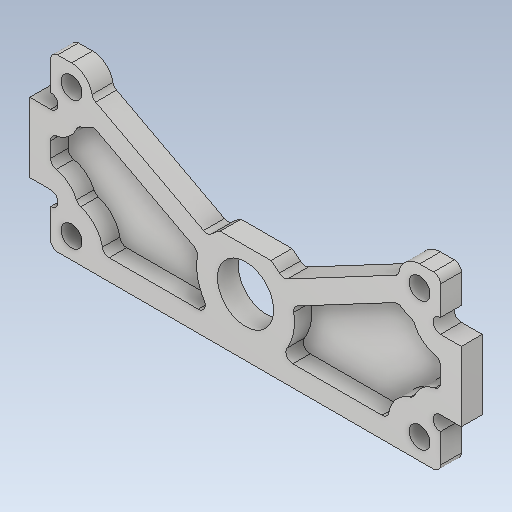
# Autodesk Inventor part: 横回転フレーム２
Saved by Autodesk Inventor 2020 (Build 240168000, 168)
## iProperties
Created: 2019-09-04
Part Number: 横回転フレーム２
Material: アルミニウム 2014-T4
Document SubType Name: Modeling
Designer: tanjihayato
Density: 2.8 g/cm^3
Appearance: サテン
Mass: 5.33751 g
Surface Area: 30.1878 cm^2
Volume: 1.90625 cm^3
Author: tanjihayato
Autodesk Inventor part; units mm, degrees
ref_plane "YZ Plane" through (0, 0, 0) normal (1, 0, 0) x (0, 1, 0)
ref_plane "XZ Plane" through (0, 0, 0) normal (0, 1, 0) x (-1, 0, 0)
ref_plane "XY Plane" through (0, 0, 0) normal (0, 0, 1) x (1, 0, 0)
sketch "スケッチ1" plane through (0, 0, 0) normal (0, 0, 1) x (1, 0, 0)
  line L0 (0, 0) -> (0, 4) construction
  line L1 (0, 0) -> (-5.3121, 14.0279)
  line L2 (-5.3121, 14.0279) -> (3.582, -2.7619)
  circle A0 centre (0.3052, 3.4238) radius 4
  line L3 (-57.3278, -140) -> (69.8706, -140)
  line L4 (0.3052, 3.4238) -> (-114.5721, -57.4302)
  circle A1 centre (0, 0) radius 23.1
  circle A2 centre (0, -29.1039) radius 6.0039
  line L5 (0, 0) -> (0, -29.1039) construction
  circle A3 centre (0, -29.1039) radius 20.05
  circle A4 centre (0, -4.0039) radius 5.05
  circle A5 centre (0, 4) radius 3
  circle A6 centre (0, -4.0039) radius 20.05
  circle A7 centre (-14, 13.4079) radius 2.2921
  circle A8 centre (14, 13.4079) radius 2.2921
  circle A9 centre (14, -21.4157) radius 2.2921
  circle A10 centre (-14, -21.4157) radius 2.2921
  circle A11 centre (-14, 13.4079) radius 14
  circle A12 centre (14, 13.4079) radius 14
  circle A13 centre (14, -21.4157) radius 14
  circle A14 centre (-14, -21.4157) radius 14
  line L6 (-14, 13.4079) -> (-14, -21.4157) construction
  line L7 (-14, -21.4157) -> (14, -21.4157) construction
  circle A15 centre (0, 0) radius 9
  line L8 (3.582, -2.7619) -> (-0.1629, 4.3075) construction
  line L9 (6.2551, -1.3458) -> (2.5102, 5.7235)
  line L10 (-2.836, 2.8915) -> (0.9089, -4.1779)
  arc A16 (0.9089, -4.1779) -> (6.2551, -1.3458) centre (3.582, -2.7619) ccw
  arc A17 (2.5102, 5.7235) -> (-2.836, 2.8915) centre (-0.1629, 4.3075) ccw
  line L11 (-5, 2.8868) -> (5, 2.8868) construction
  line L12 (5, 2.8868) -> (0, -5.7735) construction
  line L13 (0, -5.7735) -> (-5, 2.8868) construction
  circle A18 centre (-5, 2.8868) radius 1.5
  circle A19 centre (5, 2.8868) radius 1.5
  circle A20 centre (0, -5.7735) radius 1.5
  line L14 (-28, 26.018) -> (-28, -39.908)
  line L15 (28, 26.019) -> (28, -39.909)
  line L16 (-28, 29.3694) -> (28, 29.3694)
  circle A21 centre (0, 0) radius 25.1
  line L17 (-28, -18.848) -> (28, -18.848)
  circle A22 centre (0, -29.1039) radius 8.0039
  circle A23 centre (-25, 26.3694) radius 3
  circle A24 centre (25, 26.3694) radius 3
  circle A25 centre (25, -34.3772) radius 3
  circle A26 centre (-25, -34.3772) radius 3
  circle A27 centre (-25, -15.848) radius 3
  circle A28 centre (25, -15.848) radius 3
  circle A29 centre (-25, -15.848) radius 4.5
  circle A30 centre (25, -15.848) radius 4.5
  circle A31 centre (0, -4.0039) radius 4.5
  point P0 (1.7095, 0.7728)
  dimension "d0" = 4
  dimension "d1" = 15
  dimension "d2" = 11.348
  dimension "d3" = 19
  dimension "d4" = 8
  dimension "d5" = 12
  dimension "d6" = 140
  dimension "d7" = 130
  dimension "d8" = 46.2
  dimension "d9" = 29.1039
  dimension "d10" = 40.1
  dimension "d11" = 10.1
  dimension "d12" = 6
  dimension "d13" = 40.1
  dimension "d14" = 22.3421
  dimension "d15" = 22.3421
  dimension "d16" = 22.3421
  dimension "d17" = 22.3421
  dimension "d18" = 28
  dimension "d19" = 28
  dimension "d20" = 28
  dimension "d21" = 28
  dimension "d22" = 18
  dimension "d23" = 8
  dimension "d24" = 6.05
  dimension "d25" = 3
  dimension "d26" = 3
  dimension "d27" = 3
  dimension "d28" = 10
  dimension "d29" = 2
  dimension "d30" = 2
  dimension "d31" = 6
  dimension "d32" = 6
  dimension "d33" = 6
  dimension "d34" = 6
  dimension "d35" = 6
  dimension "d36" = 6
  dimension "d37" = 9
  dimension "d38" = 9
  dimension "d39" = 9
  constraints: 38 end point, 32 centre point, 28 tangent, 16 coincident, 8 point on line, 5 vertical, 4 point on circle, 3 horizontal, 3 perpendicular, 1 midpoint, 1 parallel, 7 other
  measures "d0" distance of L0.start L0.end
  measures "d1" distance of L0.start L1.end
  measures "d2" distance of L0.end L1.end
  measures "d3" distance of L1.end L2.end
  measures "d4" diameter of A0
  measures "d5" distance of L1.end L4.start
  measures "d6" distance from line of L3 L0.start
  measures "d7" distance of L4.start L4.end
  measures "d8" diameter of A1
  measures "d9" distance of L5.end L0.start
  measures "d10" diameter of A3
  measures "d11" diameter of A4
  measures "d12" diameter of A5
  measures "d13" diameter of A6
  measures "d14" distance of A7.centre A6.centre
  measures "d15" distance of A4.centre A8.centre
  measures "d16" distance of A4.centre A9.centre
  measures "d17" distance of A4.centre A10.centre
  measures "d18" diameter of A11
  measures "d19" diameter of A12
  measures "d20" diameter of A13
  measures "d21" diameter of A14
  measures "d22" diameter of A15
  measures "d23" distance of L2.end L8.end
  measures "d24" diameter of A17
  measures "d25" diameter of A18
  measures "d26" diameter of A19
  measures "d27" diameter of A20
  measures "d28" distance of L11.end L12.end
  measures "d29" radial gap between concentric circles of A1 A21
  measures "d30" radial gap between concentric circles of A2 A22
  measures "d31" diameter of A23
  measures "d32" diameter of A24
  measures "d33" diameter of A25
  measures "d34" diameter of A26
  measures "d35" diameter of A27
  measures "d36" diameter of A28
  measures "d37" diameter of A29
  measures "d38" diameter of A30
  measures "d39" diameter of A31
sketch "スケッチ2" plane through (0, 0, 0) normal (0, 0, 1) x (1, 0, 0)
  circle A0 centre (-25, -15.848) radius 3 construction
  circle A1 centre (-25, -34.3772) radius 3 construction
  circle A2 centre (25, -34.3772) radius 3 construction
  circle A3 centre (25, -15.848) radius 3 construction
  circle A4 centre (0, -29.1039) radius 20.05 construction
  circle A5 centre (-25, -15.848) radius 1.5
  circle A6 centre (25, -15.848) radius 1.5
  circle A7 centre (25, -34.3772) radius 1.5
  circle A8 centre (-25, -34.3772) radius 1.5
  circle A9 centre (0, -29.1039) radius 4.025
  line L0 (-28, -37.3772) -> (28, -37.3772)
  line L1 (28, -37.3772) -> (28, -32.2126)
  line L2 (28, -30.1126) -> (31, -30.1126)
  line L3 (31, -30.1126) -> (31, -20.1126)
  line L4 (31, -20.1126) -> (28, -20.1126)
  line L5 (28, -18.0126) -> (28, -12.848)
  line L6 (28, -12.848) -> (-28, -12.848)
  line L7 (-28, -12.848) -> (-28, -18.0126)
  line L8 (-28, -20.1126) -> (-31, -20.1126)
  line L9 (-31, -20.1126) -> (-31, -30.1126)
  line L10 (-31, -30.1126) -> (-28, -30.1126)
  line L11 (-28, -32.2126) -> (-28, -37.3772)
  arc A10 (-28, -32.2126) -> (-28, -30.1126) centre (-28, -31.1626) ccw
  arc A11 (-28, -20.1126) -> (-28, -18.0126) centre (-28, -19.0626) ccw
  arc A12 (28, -18.0126) -> (28, -20.1126) centre (28, -19.0626) ccw
  arc A13 (28, -30.1126) -> (28, -32.2126) centre (28, -31.1626) ccw
  line L12 (28, -23.1126) -> (28, -27.1126)
  arc A14 (28, -27.1126) -> (24.1322, -29.9617) centre (28, -31.1626) ccw
  line L13 (-28, -27.1126) -> (-28, -23.1126)
  arc A15 (-28, -23.1126) -> (-24.1322, -20.2636) centre (-28, -19.0626) ccw
  arc A16 (20.5, -15.848) -> (24.1322, -20.2636) centre (25, -15.848) ccw
  arc A17 (24.1322, -29.9617) -> (20.5, -34.3772) centre (25, -34.3772) ccw
  arc A18 (-20.5, -34.3772) -> (-24.1322, -29.9617) centre (-25, -34.3772) ccw
  arc A19 (-24.1322, -20.2636) -> (-20.5, -15.848) centre (-25, -15.848) ccw
  arc A20 (-24.1322, -29.9617) -> (-28, -27.1126) centre (-28, -31.1626) ccw
  arc A21 (24.1322, -20.2636) -> (28, -23.1126) centre (28, -19.0626) ccw
  arc A22 (4.6415, -34.3772) -> (-4.6415, -34.3772) centre (0, -29.1039) ccw
  line L14 (20.5, -34.3772) -> (4.6415, -34.3772)
  line L15 (-4.6415, -34.3772) -> (-20.5, -34.3772)
  line L16 (-25, -15.848) -> (0, -29.1039) construction
  arc A23 (-24.2973, -14.5228) -> (-25.7027, -17.1733) centre (-25, -15.848) ccw
  arc A24 (-0.7027, -30.4291) -> (0.7027, -27.7787) centre (0, -29.1039) ccw
  line L17 (25, -15.848) -> (0, -29.1039) construction
  arc A25 (25.7027, -17.1733) -> (24.2973, -14.5228) centre (25, -15.848) ccw
  arc A26 (-0.7027, -27.7787) -> (0.7027, -30.4291) centre (0, -29.1039) ccw
  line L18 (0.7027, -30.4291) -> (4.0026, -28.6794)
  line L19 (2.5972, -26.029) -> (-0.7027, -27.7787)
  line L20 (0.7027, -27.7787) -> (-2.5972, -26.029)
  line L21 (-4.0026, -28.6794) -> (-0.7027, -30.4291)
  line L22 (-5.3607, -24.5637) -> (-20.549, -16.5103)
  line L23 (-22.0019, -15.7399) -> (-24.2973, -14.5228)
  line L24 (-25.7027, -17.1733) -> (-23.4073, -18.3903)
  line L25 (-21.9544, -19.1607) -> (-6.766, -27.2141)
  line L26 (6.766, -27.2141) -> (21.9544, -19.1607)
  line L27 (23.4073, -18.3903) -> (25.7027, -17.1733)
  line L28 (24.2973, -14.5228) -> (21.798, -15.848)
  line L29 (20.549, -16.5103) -> (5.3607, -24.5637)
  line L30 (-20.5, -15.848) -> (20.5, -15.848)
  line L31 (21.798, -15.848) -> (22, -15.848)
  point P0 (0, 0)
  point P1 (-12.5, -22.476)
  point P2 (12.5, -22.476)
  dimension "d40" = 3
  dimension "d41" = 3
  dimension "d42" = 3
  dimension "d43" = 3
  dimension "d44" = 8.05
  dimension "d47" = 3
  dimension "d48" = 10
  dimension "d49" = 3
  dimension "d50" = 3
  dimension "d51" = 10
  dimension "d52" = 7.2646
  dimension "d53" = 7.2646
  dimension "d54" = 2.1
  dimension "d55" = 2.1
  dimension "d56" = 2.1
  dimension "d57" = 2.1
  dimension "d59" = 3
  dimension "d60" = 3
  dimension "d61" = 3
  dimension "d62" = 3
  dimension "d64" = 3
  dimension "d66" = 3
  dimension "d67" = 4.05
  dimension "d68" = 4.05
  dimension "d69" = 4.05
  dimension "d70" = 4.05
  dimension "d71" = 3
  dimension "d72" = 3
  dimension "d73" = 3
  dimension "d74" = 3
  dimension "d75" = 3
  constraints: 68 end point, 50 point on circle, 32 tangent, 22 centre point, 18 parallel, 9 point on line, 6 perpendicular, 5 coincident, 2 horizontal, 2 midpoint, 1 concentric, 1 vertical
  measures "d40" diameter of A5
  measures "d41" diameter of A6
  measures "d42" diameter of A7
  measures "d43" diameter of A8
  measures "d44" diameter of A9
  measures "d47" distance of L2.start L2.end
  measures "d48" distance of L2.end L3.end
  measures "d49" distance of L3.end L4.end
  measures "d50" distance of L8.start L8.end
  measures "d51" distance of L8.end L9.end
  measures "d52" distance between parallel lines of L4 L6
  measures "d53" distance between parallel lines of L0 L2
  measures "d54" diameter of A10
  measures "d55" diameter of A11
  measures "d56" diameter of A12
  measures "d57" diameter of A13
  measures "d59" radial gap between concentric circles of A6 A16
  measures "d60" radial gap between concentric circles of A7 A17
  measures "d61" radial gap between concentric circles of A8 A18
  measures "d62" radial gap between concentric circles of A5 A19
  measures "d64" distance between parallel lines of L3 L12
  measures "d66" distance between parallel lines of L9 L13
  measures "d67" radius of A15
  measures "d68" radius of A20
  measures "d69" radius of A14
  measures "d70" radius of A21
  measures "d71" radial gap between concentric circles of A9 A22
  measures "d72" distance between parallel lines of L0 L14
  measures "d73" distance between parallel lines of L0 L15
  measures "d74" diameter of A24
  measures "d75" diameter of A26
extrude "押し出し1" add sketch "スケッチ2" along normal blind 3 contours L11 A10 L10 L9 L8 A11 L7 L6 L5 A12 L4 L3 L2 A13 L1 L0 | L26 A22 L29 A16 | A22 L25 A19 L22
fillet "フィレット1" radius 1 22 edges at (-28, -23.1126, 1.5) (-28, -27.1126, 1.5) (-24.1322, -29.9617, 1.5) (-20.5, -34.3772, 1.5) (-4.6415, -34.3772, 1.5) (-6.766, -27.2141, 1.5) (-21.9544, -19.1607, 1.5) (-24.1322, -20.2636, 1.5) (28, -27.1126, 1.5) (28, -23.1126, 1.5) (24.1322, -20.2636, 1.5) (21.9544, -19.1607, 1.5) (6.766, -27.2141, 1.5) (4.6415, -34.3772, 1.5) (20.5, -34.3772, 1.5) (24.1322, -29.9617, 1.5) (20.5, -15.848, 1.5) (-20.5, -15.848, 1.5) (-20.549, -16.5103, 1.5) (-5.3607, -24.5637, 1.5) (5.3607, -24.5637, 1.5) (20.549, -16.5103, 1.5)
sketch "スケッチ3" plane through (0, 0, 0) normal (0, 0, -1) x (-1, 0, 0)
  line L0 (-17.7774, -15.848) -> (17.7774, -15.848) projected
  arc A0 (18.2458, -17.7315) -> (17.7774, -15.848) centre (17.7774, -16.848) ccw projected
  line L1 (18.2458, -17.7315) -> (6.0345, -24.2064) projected
  arc A1 (4.8724, -24.0433) -> (6.0345, -24.2064) centre (5.566, -23.3229) ccw projected
  arc A2 (4.8724, -24.0433) -> (-4.8724, -24.0433) centre (0, -29.1039) ccw projected
  arc A3 (-6.0345, -24.2064) -> (-4.8724, -24.0433) centre (-5.566, -23.3229) ccw projected
  line L2 (-6.0345, -24.2064) -> (-18.2458, -17.7315) projected
  arc A4 (-17.7774, -15.848) -> (-18.2458, -17.7315) centre (-17.7774, -16.848) ccw projected
  line L3 (28, -24.0126) -> (28, -26.2126) projected
  arc A5 (27.198, -27.1928) -> (28, -26.2126) centre (27, -26.2126) ccw projected
  arc A6 (27.198, -27.1928) -> (24.2958, -29.5251) centre (28, -31.1626) ccw projected
  arc A7 (23.6755, -30.0765) -> (24.2958, -29.5251) centre (23.3812, -29.1208) ccw projected
  arc A8 (23.6755, -30.0765) -> (20.575, -33.559) centre (25, -34.3772) ccw projected
  arc A9 (19.5917, -34.3772) -> (20.575, -33.559) centre (19.5917, -33.3772) ccw projected
  line L4 (19.5917, -34.3772) -> (6.7926, -34.3772) projected
  arc A10 (5.9462, -32.8447) -> (6.7926, -34.3772) centre (6.7926, -33.3772) ccw projected
  arc A11 (5.9462, -32.8447) -> (6.9228, -27.9103) centre (0, -29.1039) ccw projected
  arc A12 (7.4399, -26.8568) -> (6.9228, -27.9103) centre (7.9083, -27.7403) ccw projected
  line L5 (7.4399, -26.8568) -> (21.3745, -19.4682) projected
  arc A13 (22.417, -19.5329) -> (21.3745, -19.4682) centre (21.843, -20.3517) ccw projected
  arc A14 (22.417, -19.5329) -> (23.6755, -20.1487) centre (25, -15.848) ccw projected
  arc A15 (24.2958, -20.7001) -> (23.6755, -20.1487) centre (23.3812, -21.1044) ccw projected
  arc A16 (24.2958, -20.7001) -> (27.198, -23.0324) centre (28, -19.0626) ccw projected
  arc A17 (28, -24.0126) -> (27.198, -23.0324) centre (27, -24.0126) ccw projected
  line L6 (-28, -26.2126) -> (-28, -24.0126) projected
  arc A18 (-27.198, -23.0324) -> (-28, -24.0126) centre (-27, -24.0126) ccw projected
  arc A19 (-27.198, -23.0324) -> (-24.2958, -20.7001) centre (-28, -19.0626) ccw projected
  arc A20 (-23.6755, -20.1487) -> (-24.2958, -20.7001) centre (-23.3812, -21.1044) ccw projected
  arc A21 (-23.6755, -20.1487) -> (-22.417, -19.5329) centre (-25, -15.848) ccw projected
  arc A22 (-21.3745, -19.4682) -> (-22.417, -19.5329) centre (-21.843, -20.3517) ccw projected
  line L7 (-21.3745, -19.4682) -> (-7.4399, -26.8568) projected
  arc A23 (-6.9228, -27.9103) -> (-7.4399, -26.8568) centre (-7.9083, -27.7403) ccw projected
  arc A24 (-6.9228, -27.9103) -> (-5.9462, -32.8447) centre (0, -29.1039) ccw projected
  arc A25 (-6.7926, -34.3772) -> (-5.9462, -32.8447) centre (-6.7926, -33.3772) ccw projected
  line L8 (-6.7926, -34.3772) -> (-19.5917, -34.3772) projected
  arc A26 (-20.575, -33.559) -> (-19.5917, -34.3772) centre (-19.5917, -33.3772) ccw projected
  arc A27 (-20.575, -33.559) -> (-23.6755, -30.0765) centre (-25, -34.3772) ccw projected
  arc A28 (-24.2958, -29.5251) -> (-23.6755, -30.0765) centre (-23.3812, -29.1208) ccw projected
  arc A29 (-24.2958, -29.5251) -> (-27.198, -27.1928) centre (-28, -31.1626) ccw projected
  arc A30 (-28, -26.2126) -> (-27.198, -27.1928) centre (-27, -26.2126) ccw projected
  circle A31 centre (0, -29.1039) radius 4.025 projected
  line L9 (-28, -37.3772) -> (28, -37.3772) projected
  line L10 (28, -37.3772) -> (28, -32.2126) projected
  arc A32 (28, -30.1126) -> (28, -32.2126) centre (28, -31.1626) ccw projected
  line L11 (28, -30.1126) -> (31, -30.1126) projected
  line L12 (31, -30.1126) -> (31, -20.1126) projected
  line L13 (31, -20.1126) -> (28, -20.1126) projected
  arc A33 (28, -18.0126) -> (28, -20.1126) centre (28, -19.0626) ccw projected
  line L14 (28, -18.0126) -> (28, -12.848) projected
  line L15 (28, -12.848) -> (-28, -12.848) projected
  line L16 (-28, -12.848) -> (-28, -18.0126) projected
  arc A34 (-28, -20.1126) -> (-28, -18.0126) centre (-28, -19.0626) ccw projected
  line L17 (-28, -20.1126) -> (-31, -20.1126) projected
  line L18 (-31, -20.1126) -> (-31, -30.1126) projected
  line L19 (-31, -30.1126) -> (-28, -30.1126) projected
  arc A35 (-28, -32.2126) -> (-28, -30.1126) centre (-28, -31.1626) ccw projected
  line L20 (-28, -32.2126) -> (-28, -37.3772) projected
  circle A36 centre (25, -15.848) radius 1.5 projected
  circle A37 centre (-25, -15.848) radius 1.5 projected
  circle A38 centre (-25, -34.3772) radius 1.5 projected
  circle A39 centre (25, -34.3772) radius 1.5 projected
  point P0 (0, 0)
extrude "押し出し2" add sketch "スケッチ3" against normal blind 0.5 contours L0 A0 L1 A1 A2 A3 L2 A4 | L3 A5 A6 A7 A8 A9 L4 A10 A11 A12 L5 A13 A14 A15 A16 A17 | L6 A18 A19 A20 A21 A22 L7 A23 A24 A25 L8 A26 A27 A28 A29 A30
sketch "スケッチ4" plane through (0, 0, 3) normal (0, 0, 1) x (1, 0, 0)
  line L0 (-17.7774, -15.848) -> (17.7774, -15.848) projected
  arc A0 (18.2458, -17.7315) -> (17.7774, -15.848) centre (17.7774, -16.848) ccw projected
  line L1 (18.2458, -17.7315) -> (6.0345, -24.2064) projected
  arc A1 (4.8724, -24.0433) -> (6.0345, -24.2064) centre (5.566, -23.3229) ccw projected
  arc A2 (4.8724, -24.0433) -> (-4.8724, -24.0433) centre (0, -29.1039) ccw projected
  arc A3 (-6.0345, -24.2064) -> (-4.8724, -24.0433) centre (-5.566, -23.3229) ccw projected
  line L2 (-6.0345, -24.2064) -> (-18.2458, -17.7315) projected
  arc A4 (-17.7774, -15.848) -> (-18.2458, -17.7315) centre (-17.7774, -16.848) ccw projected
  line L3 (-28, -26.2126) -> (-28, -24.0126) projected
  arc A5 (-27.198, -23.0324) -> (-28, -24.0126) centre (-27, -24.0126) ccw projected
  arc A6 (-27.198, -23.0324) -> (-24.2958, -20.7001) centre (-28, -19.0626) ccw projected
  arc A7 (-23.6755, -20.1487) -> (-24.2958, -20.7001) centre (-23.3812, -21.1044) ccw projected
  arc A8 (-23.6755, -20.1487) -> (-22.417, -19.5329) centre (-25, -15.848) ccw projected
  arc A9 (-21.3745, -19.4682) -> (-22.417, -19.5329) centre (-21.843, -20.3517) ccw projected
  line L4 (-21.3745, -19.4682) -> (-7.4399, -26.8568) projected
  arc A10 (-6.9228, -27.9103) -> (-7.4399, -26.8568) centre (-7.9083, -27.7403) ccw projected
  arc A11 (-6.9228, -27.9103) -> (-5.9462, -32.8447) centre (0, -29.1039) ccw projected
  arc A12 (-6.7926, -34.3772) -> (-5.9462, -32.8447) centre (-6.7926, -33.3772) ccw projected
  line L5 (-6.7926, -34.3772) -> (-19.5917, -34.3772) projected
  arc A13 (-20.575, -33.559) -> (-19.5917, -34.3772) centre (-19.5917, -33.3772) ccw projected
  arc A14 (-20.575, -33.559) -> (-23.6755, -30.0765) centre (-25, -34.3772) ccw projected
  arc A15 (-24.2958, -29.5251) -> (-23.6755, -30.0765) centre (-23.3812, -29.1208) ccw projected
  arc A16 (-24.2958, -29.5251) -> (-27.198, -27.1928) centre (-28, -31.1626) ccw projected
  arc A17 (-28, -26.2126) -> (-27.198, -27.1928) centre (-27, -26.2126) ccw projected
  line L6 (28, -24.0126) -> (28, -26.2126) projected
  arc A18 (27.198, -27.1928) -> (28, -26.2126) centre (27, -26.2126) ccw projected
  arc A19 (27.198, -27.1928) -> (24.2958, -29.5251) centre (28, -31.1626) ccw projected
  arc A20 (23.6755, -30.0765) -> (24.2958, -29.5251) centre (23.3812, -29.1208) ccw projected
  arc A21 (23.6755, -30.0765) -> (20.575, -33.559) centre (25, -34.3772) ccw projected
  arc A22 (19.5917, -34.3772) -> (20.575, -33.559) centre (19.5917, -33.3772) ccw projected
  line L7 (19.5917, -34.3772) -> (6.7926, -34.3772) projected
  arc A23 (5.9462, -32.8447) -> (6.7926, -34.3772) centre (6.7926, -33.3772) ccw projected
  arc A24 (5.9462, -32.8447) -> (6.9228, -27.9103) centre (0, -29.1039) ccw projected
  arc A25 (7.4399, -26.8568) -> (6.9228, -27.9103) centre (7.9083, -27.7403) ccw projected
  line L8 (7.4399, -26.8568) -> (21.3745, -19.4682) projected
  arc A26 (22.417, -19.5329) -> (21.3745, -19.4682) centre (21.843, -20.3517) ccw projected
  arc A27 (22.417, -19.5329) -> (23.6755, -20.1487) centre (25, -15.848) ccw projected
  arc A28 (24.2958, -20.7001) -> (23.6755, -20.1487) centre (23.3812, -21.1044) ccw projected
  arc A29 (24.2958, -20.7001) -> (27.198, -23.0324) centre (28, -19.0626) ccw projected
  arc A30 (28, -24.0126) -> (27.198, -23.0324) centre (27, -24.0126) ccw projected
  line L9 (-28, -37.3772) -> (28, -37.3772) projected
  line L10 (28, -37.3772) -> (28, -32.2126) projected
  arc A31 (28, -30.1126) -> (28, -32.2126) centre (28, -31.1626) ccw projected
  line L11 (28, -30.1126) -> (31, -30.1126) projected
  line L12 (31, -30.1126) -> (31, -20.1126) projected
  line L13 (31, -20.1126) -> (28, -20.1126) projected
  arc A32 (28, -18.0126) -> (28, -20.1126) centre (28, -19.0626) ccw projected
  line L14 (28, -18.0126) -> (28, -12.848) projected
  line L15 (28, -12.848) -> (-28, -12.848) projected
  line L16 (-28, -12.848) -> (-28, -18.0126) projected
  arc A33 (-28, -20.1126) -> (-28, -18.0126) centre (-28, -19.0626) ccw projected
  line L17 (-28, -20.1126) -> (-31, -20.1126) projected
  line L18 (-31, -20.1126) -> (-31, -30.1126) projected
  line L19 (-31, -30.1126) -> (-28, -30.1126) projected
  arc A34 (-28, -32.2126) -> (-28, -30.1126) centre (-28, -31.1626) ccw projected
  line L20 (-28, -32.2126) -> (-28, -37.3772) projected
  circle A35 centre (-25, -15.848) radius 1.5 projected
  circle A36 centre (25, -15.848) radius 1.5 projected
  circle A37 centre (25, -34.3772) radius 1.5 projected
  circle A38 centre (-25, -34.3772) radius 1.5 projected
  circle A39 centre (0, -29.1039) radius 4.025 projected
  arc A40 (-22.0019, -15.7399) -> (-25, -12.848) centre (-25, -15.848) ccw
  arc A41 (25, -12.848) -> (22.0019, -15.7399) centre (25, -15.848) ccw
  line L21 (-18.2458, -17.7315) -> (-22.0019, -15.7399)
  line L22 (18.2458, -17.7315) -> (22.0019, -15.7399)
  line L23 (18.2458, -17.7315) -> (6.0345, -24.2064) projected
  line L24 (-6.0345, -24.2064) -> (-18.2458, -17.7315) projected
  line L25 (-3.6539, -23.1039) -> (3.6539, -23.1039)
  point P0 (0, 0)
  dimension "d81" = 6
  dimension "d82" = 6
  dimension "d83" = 6
  constraints: 6 end point, 6 point on circle, 2 centre point, 2 coincident, 2 collinear, 2 point on line, 1 horizontal
  measures "d81" diameter of A40
  measures "d82" diameter of A41
  measures "d83" distance from line of A2.centre L25
extrude "押し出し3" cut sketch "スケッチ4" against normal blind 3 contours A4 L21 A40 L15 A41 L22 A0 L0 | L0 A0 L1 A1 A2 A3 L2 A4 | A2 L25
fillet "フィレット2" radius 1 2 edges at (-22.0019, -15.7399, 1.5) (22.0019, -15.7399, 1.5)
fillet "フィレット3" radius 1 4 edges at (-28, -12.848, 1.5) (28, -12.848, 1.5) (28, -37.3772, 1.5) (-28, -37.3772, 1.5)
equation "\"d15\" = d14"
equation "\"d16\" = d14"
equation "\"d17\" = d14"
equation "\"d53\" = d52"
